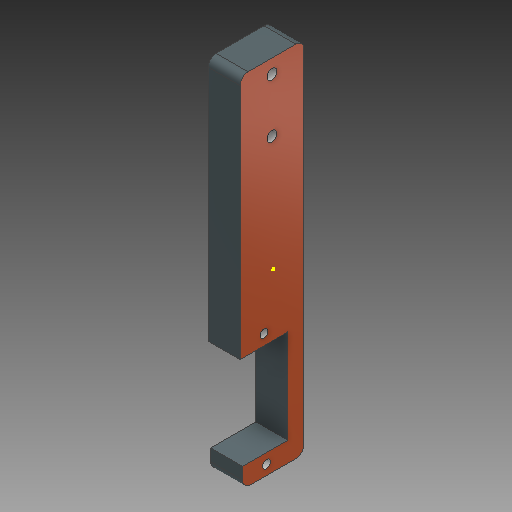
# Autodesk Inventor part: Arm1
Saved by Autodesk Inventor 2018 (Build 220112000, 112)
## iProperties
Created: 2018-09-18
Part Number: Arm1
Material: Generic
Document SubType Name: Modeling
Designer: Viraj Shah
Density: 1 g/cm^3
Appearance: Default
Mass: 9.08212 g
Surface Area: 43.4701 cm^2
Volume: 9.08212 cm^3
Author: Viraj Shah
Autodesk Inventor part; units mm, degrees
ref_plane "YZ Plane" through (0, 0, 0) normal (1, 0, 0) x (0, 1, 0)
ref_plane "XZ Plane" through (0, 0, 0) normal (0, 1, 0) x (-1, 0, 0)
ref_plane "XY Plane" through (0, 0, 0) normal (0, 0, 1) x (1, 0, 0)
sketch "Sketch1" plane through (0, 0, 0) normal (1, 0, 0) x (0, 1, 0)
  line L0 (-7.5231, -44.0814) -> (7.8367, -44.0814)
  line L1 (7.8367, -44.0814) -> (7.8367, 45.9186)
  line L2 (7.8367, 45.9186) -> (-8.1633, 45.9186)
  line L3 (-7.5231, -44.0814) -> (7.8367, 45.9186) construction
  line L4 (7.8367, -44.0814) -> (-8.1633, 45.9186) construction
  line L5 (-8.1633, 45.9186) -> (-8.1633, -15.5814)
  line L6 (3.8367, -15.5814) -> (-8.1633, -15.5814)
  line L7 (3.8367, -15.5814) -> (3.8367, -39.0814)
  line L8 (3.8367, -39.0814) -> (-7.5231, -39.0814)
  line L9 (-7.5231, -39.0814) -> (-7.5231, -44.0814)
  point P0 (0, 0)
  dimension "d0" = 16
  dimension "d1" = 90
  dimension "d24" = 12
  dimension "d28" = 5
  dimension "d29" = 23.5
  constraints: 20 end point, 3 horizontal, 2 parallel, 2 perpendicular, 2 point on line, 1 vertical
  measures "d0" distance of L1.end L2.end
  measures "d1" distance of L0.end L1.end
  measures "d24" distance of L5.end L6.start
  measures "d28" distance of L8.end L0.start
  measures "d29" distance between parallel lines of L8 L6
extrude "Extrusion1" add sketch "Sketch1" along normal blind 8
sketch "Sketch2" plane through (8, 0, 0) normal (1, 0, 0) x (0, 0, -1)
  point P0 (0, 0)
sketch "Sketch3" plane through (8, 0, 0) normal (1, 0, 0) x (0, 0, -1)
  line L0 (-45.9186, 7.8367) -> (-45.9186, -8.1633) projected
  line L1 (44.0814, -7.5231) -> (44.0814, 7.8367) projected
  point P0 (0, 0)
  point P1 (-28.9186, -0.1633)
  point P2 (27.0814, 0.4769)
  point P3 (-42.4186, -0.1633)
  dimension "d4" = 17
  dimension "d5" = 17
  dimension "d23" = 13.5
  measures "d4" distance from line of point (-28.919, -0.163) L0
  measures "d5" distance from line of L1 point (27.081, 0.477)
  measures "d23" distance of point (-28.919, -0.163) point (-42.419, -0.163)
hole "Hole1" at (8, -0.1633, 28.9186) at (8, -0.1633, 42.4186) direction (-1, 0, 0) diameter 2.5 end through all
fillet "Fillet1" radius 2 4 edges at (4, 7.8367, 45.9186) (4, -8.1633, 45.9186) (4, 7.8367, -44.0814) (4, -7.5231, -44.0814)
sketch "Sketch4" plane through (8, 0, 0) normal (1, 0, 0) x (0, 0, -1)
  line L0 (44.0814, -5.5231) -> (44.0814, 5.8367) projected
  line L1 (-43.9186, -8.1633) -> (15.5814, -8.1633) projected
  line L2 (39.0814, -7.5231) -> (42.0814, -7.5231) projected
  point P0 (0, 0)
  point P1 (41.5814, -1.5231)
  point P2 (12.8885, -2.1633)
  dimension "d14" = 2.5
  dimension "d15" = 28.7
  dimension "d30" = 6
  dimension "d31" = 6
  measures "d14" distance from line of L0 point (41.581, -1.523)
  measures "d15" distance of point (41.581, -1.523) point (12.889, -2.163)
  measures "d30" distance from line of L1 point (12.889, -2.163)
  measures "d31" distance from line of L2 point (41.581, -1.523)
hole "Hole2" at (8, -2.1633, -12.8885) at (8, -1.5231, -41.5814) direction (-1, 0, 0) diameter 2 end through all
body "Solid1"
